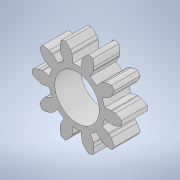
# Autodesk Inventor part: m1歯数10ギア3.5t
Saved by Autodesk Inventor 2020.2 (Build 242310000, 310)
## iProperties
Created: 2020-02-29
Part Number: m1歯数10ギア3.5t
Material: 一般
Document SubType Name: Modeling
Designer: aoyam
Density: 1 g/cm^3
Appearance: 既定
Author: aoyam
Autodesk Inventor part; units mm, degrees
ref_plane "YZ Plane" through (0, 0, 0) normal (1, 0, 0) x (0, 1, 0)
ref_plane "XZ Plane" through (0, 0, 0) normal (0, 1, 0) x (-1, 0, 0)
ref_plane "XY Plane" through (0, 0, 0) normal (0, 0, 1) x (1, 0, 0)
sketch "スケッチ1" plane through (0, 0, 0) normal (0, 0, 1) x (1, 0, 0)
  arc A0 (1.8273, 5.9318) -> (1.7922, 5.8155) centre (2.3801, 5.701) ccw
  arc A1 (2.032, 6.2968) -> (1.8273, 5.9318) centre (3.3772, 5.3028) ccw
  arc A2 (2.6989, 6.9547) -> (2.032, 6.2968) centre (4.4405, 4.5224) ccw
  arc A3 (0.4607, 5.8155) -> (0.4255, 5.9318) centre (-0.1273, 5.701) ccw
  arc A4 (0.4255, 5.9318) -> (0.2209, 6.2968) centre (-1.1244, 5.3028) ccw
  arc A5 (0.2209, 6.2968) -> (-0.4461, 6.9547) centre (-2.1876, 4.5224) ccw
  arc A6 (1.6578, 4.8766) -> (0.595, 4.8766) centre (1.1264, 1.1645) ccw
  arc A7 (-0.4461, 6.9547) -> (-1.0048, 6.7732) centre (1.1264, 1.1645) ccw
  line L0 (1.6578, 4.8766) -> (1.7922, 5.8155)
  line L1 (0.595, 4.8766) -> (0.4607, 5.8155)
  line L2 (-6.8736, 1.1645) -> (9.1264, 1.1645)
  arc A8 (-2.146, 4.5359) -> (-2.2428, 4.6093) centre (-2.5544, 4.0977) ccw
  arc A9 (-2.2428, 4.6093) -> (-2.6229, 4.7843) centre (-3.127, 3.1894) ccw
  arc A10 (-2.6229, 4.7843) -> (-3.5492, 4.9246) centre (-3.5284, 1.9331) ccw
  arc A11 (-3.5492, 4.9246) -> (-3.8945, 4.4493) centre (1.1264, 1.1645) ccw
  line L3 (-1.4854, 3.8553) -> (-2.146, 4.5359)
  arc A12 (-0.6257, 4.48) -> (-1.4854, 3.8553) centre (1.1264, 1.1645) ccw
  line L4 (-0.6257, 4.48) -> (-1.0688, 5.3186)
  arc A13 (-1.1087, 5.4333) -> (-1.0688, 5.3186) centre (-0.5258, 5.5715) ccw
  arc A14 (-1.1577, 5.8488) -> (-1.1087, 5.4333) centre (0.5149, 5.8354) ccw
  arc A15 (-1.0048, 6.7732) -> (-1.1577, 5.8488) centre (1.8338, 5.829) ccw
  arc A16 (-3.5027, 1.9686) -> (-3.6242, 1.971) centre (-3.5755, 1.374) ccw
  arc A17 (-3.6242, 1.971) -> (-4.0345, 1.8892) centre (-3.5049, 0.3026) ccw
  arc A18 (-4.0345, 1.8892) -> (-4.8664, 1.4582) centre (-3.0912, -0.9497) ccw
  arc A19 (-4.8664, 1.4582) -> (-4.8664, 0.8707) centre (1.1264, 1.1645) ccw
  line L5 (-2.5683, 1.8062) -> (-3.5027, 1.9686)
  arc A20 (-2.2399, 2.817) -> (-2.5683, 1.8062) centre (1.1264, 1.1645) ccw
  line L6 (-2.2399, 2.817) -> (-3.0913, 3.2349)
  arc A21 (-3.191, 3.3043) -> (-3.0913, 3.2349) centre (-2.8007, 3.7587) ccw
  arc A22 (-3.4749, 3.6117) -> (-3.191, 3.3043) centre (-2.1138, 4.5839) ccw
  arc A23 (-3.8945, 4.4493) -> (-3.4749, 3.6117) centre (-1.0431, 5.354) ccw
  arc A24 (-3.0913, -0.906) -> (-3.191, -0.9753) centre (-2.8007, -1.4298) ccw
  arc A25 (-3.191, -0.9753) -> (-3.4749, -1.2827) centre (-2.1138, -2.255) ccw
  arc A26 (-3.4749, -1.2827) -> (-3.8945, -2.1204) centre (-1.0431, -3.025) ccw
  arc A27 (-3.8945, -2.1204) -> (-3.5492, -2.5956) centre (1.1264, 1.1645) ccw
  line L7 (-2.2399, -0.488) -> (-3.0913, -0.906)
  arc A28 (-2.5683, 0.5227) -> (-2.2399, -0.488) centre (1.1264, 1.1645) ccw
  line L8 (-2.5683, 0.5227) -> (-3.5027, 0.3604)
  arc A29 (-3.6242, 0.3579) -> (-3.5027, 0.3604) centre (-3.5755, 0.955) ccw
  arc A30 (-4.0345, 0.4397) -> (-3.6242, 0.3579) centre (-3.5049, 2.0263) ccw
  arc A31 (-4.8664, 0.8707) -> (-4.0345, 0.4397) centre (-3.0912, 3.2787) ccw
  arc A32 (-1.0688, -2.9896) -> (-1.1087, -3.1044) centre (-0.5258, -3.2426) ccw
  arc A33 (-1.1087, -3.1044) -> (-1.1577, -3.5199) centre (0.5149, -3.5065) ccw
  arc A34 (-1.1577, -3.5199) -> (-1.0048, -4.4443) centre (1.8338, -3.5001) ccw
  arc A35 (-1.0048, -4.4443) -> (-0.4461, -4.6258) centre (1.1264, 1.1645) ccw
  line L9 (-0.6257, -2.1511) -> (-1.0688, -2.9896)
  arc A36 (-1.4854, -1.5264) -> (-0.6257, -2.1511) centre (1.1264, 1.1645) ccw
  line L10 (-1.4854, -1.5264) -> (-2.146, -2.207)
  arc A37 (-2.2428, -2.2804) -> (-2.146, -2.207) centre (-2.5544, -1.7688) ccw
  arc A38 (-2.6229, -2.4554) -> (-2.2428, -2.2804) centre (-3.127, -0.8605) ccw
  arc A39 (-3.5492, -2.5956) -> (-2.6229, -2.4554) centre (-3.5284, 0.3958) ccw
  arc A40 (1.7922, -3.4866) -> (1.8273, -3.6028) centre (2.3801, -3.3721) ccw
  arc A41 (1.8273, -3.6028) -> (2.032, -3.9678) centre (3.3772, -2.9738) ccw
  arc A42 (2.032, -3.9678) -> (2.6989, -4.6258) centre (4.4405, -2.1934) ccw
  arc A43 (2.6989, -4.6258) -> (3.2577, -4.4443) centre (1.1264, 1.1645) ccw
  line L11 (1.6578, -2.5477) -> (1.7922, -3.4866)
  arc A44 (0.595, -2.5477) -> (1.6578, -2.5477) centre (1.1264, 1.1645) ccw
  line L12 (0.595, -2.5477) -> (0.4607, -3.4866)
  arc A45 (0.4255, -3.6028) -> (0.4607, -3.4866) centre (-0.1273, -3.3721) ccw
  arc A46 (0.2209, -3.9678) -> (0.4255, -3.6028) centre (-1.1244, -2.9738) ccw
  arc A47 (-0.4461, -4.6258) -> (0.2209, -3.9678) centre (-2.1876, -2.1934) ccw
  arc A48 (4.3988, -2.207) -> (4.4956, -2.2804) centre (4.8072, -1.7688) ccw
  arc A49 (4.4956, -2.2804) -> (4.8757, -2.4554) centre (5.3798, -0.8605) ccw
  arc A50 (4.8757, -2.4554) -> (5.802, -2.5956) centre (5.7813, 0.3958) ccw
  arc A51 (5.802, -2.5956) -> (6.1473, -2.1204) centre (1.1264, 1.1645) ccw
  line L13 (3.7382, -1.5264) -> (4.3988, -2.207)
  arc A52 (2.8785, -2.1511) -> (3.7382, -1.5264) centre (1.1264, 1.1645) ccw
  line L14 (2.8785, -2.1511) -> (3.3216, -2.9896)
  arc A53 (3.3615, -3.1044) -> (3.3216, -2.9896) centre (2.7787, -3.2426) ccw
  arc A54 (3.4105, -3.5199) -> (3.3615, -3.1044) centre (1.7379, -3.5065) ccw
  arc A55 (3.2577, -4.4443) -> (3.4105, -3.5199) centre (0.419, -3.5001) ccw
  arc A56 (5.7556, 0.3604) -> (5.877, 0.3579) centre (5.8284, 0.955) ccw
  arc A57 (5.877, 0.3579) -> (6.2873, 0.4397) centre (5.7577, 2.0263) ccw
  arc A58 (6.2873, 0.4397) -> (7.1192, 0.8707) centre (5.3441, 3.2787) ccw
  arc A59 (7.1192, 0.8707) -> (7.1192, 1.4582) centre (1.1264, 1.1645) ccw
  line L15 (4.8211, 0.5227) -> (5.7556, 0.3604)
  arc A60 (4.4927, -0.488) -> (4.8211, 0.5227) centre (1.1264, 1.1645) ccw
  line L16 (4.4927, -0.488) -> (5.3441, -0.906)
  arc A61 (5.4438, -0.9753) -> (5.3441, -0.906) centre (5.0535, -1.4298) ccw
  arc A62 (5.7277, -1.2827) -> (5.4438, -0.9753) centre (4.3666, -2.255) ccw
  arc A63 (6.1473, -2.1204) -> (5.7277, -1.2827) centre (3.2959, -3.025) ccw
  arc A64 (5.3441, 3.2349) -> (5.4438, 3.3043) centre (5.0535, 3.7587) ccw
  arc A65 (5.4438, 3.3043) -> (5.7277, 3.6117) centre (4.3666, 4.5839) ccw
  arc A66 (5.7277, 3.6117) -> (6.1473, 4.4493) centre (3.2959, 5.354) ccw
  arc A67 (6.1473, 4.4493) -> (5.802, 4.9246) centre (1.1264, 1.1645) ccw
  line L17 (4.4927, 2.817) -> (5.3441, 3.2349)
  arc A68 (4.8211, 1.8062) -> (4.4927, 2.817) centre (1.1264, 1.1645) ccw
  line L18 (4.8211, 1.8062) -> (5.7556, 1.9686)
  arc A69 (5.877, 1.971) -> (5.7556, 1.9686) centre (5.8284, 1.374) ccw
  arc A70 (6.2873, 1.8892) -> (5.877, 1.971) centre (5.7577, 0.3026) ccw
  arc A71 (7.1192, 1.4582) -> (6.2873, 1.8892) centre (5.3441, -0.9497) ccw
  arc A72 (3.3216, 5.3186) -> (3.3615, 5.4333) centre (2.7787, 5.5715) ccw
  arc A73 (3.3615, 5.4333) -> (3.4105, 5.8488) centre (1.7379, 5.8354) ccw
  arc A74 (3.4105, 5.8488) -> (3.2577, 6.7732) centre (0.419, 5.829) ccw
  arc A75 (3.2577, 6.7732) -> (2.6989, 6.9547) centre (1.1264, 1.1645) ccw
  line L19 (2.8785, 4.48) -> (3.3216, 5.3186)
  arc A76 (3.7382, 3.8553) -> (2.8785, 4.48) centre (1.1264, 1.1645) ccw
  line L20 (3.7382, 3.8553) -> (4.3988, 4.5359)
  arc A77 (4.4956, 4.6093) -> (4.3988, 4.5359) centre (4.8072, 4.0977) ccw
  arc A78 (4.8757, 4.7843) -> (4.4956, 4.6093) centre (5.3798, 3.1894) ccw
  arc A79 (5.802, 4.9246) -> (4.8757, 4.7843) centre (5.7813, 1.9331) ccw
  circle A80 centre (1.1264, 1.1645) radius 3
  point P0 (0, 0)
  point P1 (-4.0295, 1.8909)
  point P2 (-4.8664, 1.4582)
  point P3 (-4.8664, 0.8707)
  point P4 (-4.0295, 0.4381)
  point P5 (-3.6149, 0.3572)
  point P6 (-3.0913, -0.906)
  point P7 (-3.1839, -0.9694)
  point P8 (-3.4718, -1.2784)
  point P9 (-3.8945, -2.1204)
  point P10 (-3.5492, -2.5956)
  point P11 (-2.6178, -2.4538)
  point P12 (-2.235, -2.2755)
  point P13 (-1.4854, -1.5264)
  point P14 (-0.6257, -2.1511)
  point P15 (-1.1065, -3.0954)
  point P16 (-1.1577, -3.5146)
  point P17 (-1.0048, -4.4443)
  point P18 (-0.4461, -4.6258)
  point P19 (0.224, -3.9636)
  point P20 (0.429, -3.5943)
  point P21 (0.595, -2.5477)
  point P22 (1.6578, -2.5477)
  point P23 (1.8239, -3.5943)
  point P24 (2.0288, -3.9636)
  point P25 (2.6989, -4.6258)
  point P26 (3.2577, -4.4443)
  point P27 (3.4105, -3.5146)
  point P28 (3.3593, -3.0954)
  point P29 (2.8785, -2.1511)
  point P30 (4.4878, -2.2755)
  point P31 (4.8707, -2.4538)
  point P32 (5.802, -2.5956)
  point P33 (6.1473, -2.1204)
  point P34 (5.7246, -1.2784)
  point P35 (5.4367, -0.9694)
  point P36 (5.3441, -0.906)
  point P37 (4.4927, -0.488)
  point P38 (4.8211, 0.5227)
  point P39 (5.8678, 0.3572)
  point P40 (6.2823, 0.4381)
  point P41 (7.1192, 0.8707)
  point P42 (7.1192, 1.4582)
  point P43 (6.2823, 1.8909)
  point P44 (5.8678, 1.9717)
  point P45 (4.8211, 1.8062)
  point P46 (5.4367, 3.2983)
  point P47 (5.7246, 3.6074)
  point P48 (6.1473, 4.4493)
  point P49 (5.802, 4.9246)
  point P50 (4.8707, 4.7827)
  point P51 (4.4878, 4.6044)
  point P52 (3.7382, 3.8553)
  point P53 (3.3216, 5.3186)
  point P54 (3.3593, 5.4243)
  point P55 (3.4105, 5.8436)
  point P56 (3.2577, 6.7732)
  point P57 (2.6989, 6.9547)
  point P58 (2.0288, 6.2925)
  point P59 (1.8239, 5.9232)
  point P60 (1.6578, 4.8766)
  point P61 (0.595, 4.8766)
  point P62 (0.4607, 5.8155)
  point P63 (0.429, 5.9232)
  point P64 (0.224, 6.2925)
  point P65 (-0.4461, 6.9547)
  point P66 (-1.0048, 6.7732)
  point P67 (-1.1577, 5.8436)
  point P68 (-1.1065, 5.4243)
  point P69 (-0.6257, 4.48)
  point P70 (-1.4854, 3.8553)
  point P71 (-2.235, 4.6044)
  point P72 (-2.6178, 4.7827)
  point P73 (-3.5492, 4.9246)
  point P74 (-3.8945, 4.4493)
  point P75 (-3.4718, 3.6074)
  point P76 (-3.1839, 3.2983)
  point P77 (-2.5683, 1.8062)
  point P78 (-3.5027, 1.9686)
  point P79 (-3.6149, 1.9717)
  point P80 (1.8273, -3.6028)
  point P81 (2.032, -3.9678)
  point P82 (3.4105, -3.5146)
  point P83 (3.3615, -3.1044)
  point P84 (4.4956, -2.2804)
  point P85 (4.8757, -2.4554)
  point P86 (5.7277, -1.2827)
  point P87 (5.4438, -0.9753)
  point P88 (5.8678, 0.3572)
  point P89 (6.2873, 0.4397)
  point P90 (6.2823, 1.8909)
  point P91 (5.877, 1.971)
  point P92 (5.4438, 3.3043)
  point P93 (5.7246, 3.6074)
  point P94 (4.8757, 4.7843)
  point P95 (4.4956, 4.6093)
  point P96 (3.3615, 5.4333)
  point P97 (3.4105, 5.8488)
  point P98 (2.032, 6.2968)
  point P99 (1.8273, 5.9318)
  point P100 (0.4255, 5.9318)
  point P101 (0.2209, 6.2968)
  point P102 (-1.1577, 5.8436)
  point P103 (-1.1087, 5.4333)
  point P104 (-2.2428, 4.6093)
  point P105 (-2.6229, 4.7843)
  point P106 (-3.4749, 3.6117)
  point P107 (-3.1839, 3.2983)
  point P108 (-3.6149, 1.9717)
  point P109 (-4.0345, 1.8892)
  point P110 (-4.0345, 0.4397)
  point P111 (-3.6242, 0.3579)
  point P112 (-3.191, -0.9753)
  point P113 (-3.4749, -1.2827)
  point P114 (-2.6229, -2.4554)
  point P115 (-2.2428, -2.2804)
  point P116 (-1.1087, -3.1044)
  point P117 (-1.1577, -3.5199)
  point P118 (0.2209, -3.9678)
  point P119 (0.429, -3.5943)
  point P120 (0.4255, -3.6028)
  point P121 (3.4105, -3.5199)
  point P122 (5.877, 0.3579)
  point P123 (6.2873, 1.8892)
  point P124 (5.7277, 3.6117)
  point P125 (-1.1577, 5.8488)
  point P126 (-3.191, 3.3043)
  point P127 (-3.6242, 1.971)
  dimension "d2" = 360
  dimension "d12" = 6
  constraints: 160 point on circle, 81 centre point, 42 end point, 3 coincident, 379 other
  measures "d12" diameter of A80
extrude "押し出し1" add sketch "スケッチ1" along normal blind 3.5 contours A1 A2 A75 A74 A73 A72 L19 A76 L20 A77 A78 A79 A67 A66 A65 A64 L17 A68 L18 A69 A70 A71 A59 L2 A80 A19 A18 A17 A16 L5 A20 L6 A21 A22 A23 A11 A10 A9 A8 L3 A12 L4 A13 A14 A15 A7 A5 A4 A3 L1 A6 L0 A0 | A59 A58 A57 A56 L15 A60 L16 A61 A62 A63 A51 A50 A49 A48 L13 A52 L14 A53 A54 A55 A43 A42 A41 A40 L11 A44 L12 A45 A46 A47 A35 A34 A33 A32 L9 A36 L10 A37 A38 A39 A27 A26 A25 A24 L7 A28 L8 A29 A30 A31 A19 L2 A80
